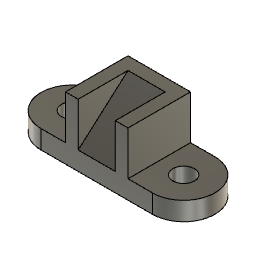
Homework - A2 (Autodesk Fusion 360 design; units mm, degrees)
Autodesk Fusion 360 part; units mm, degrees
sketch "Sketch1" plane through (0, 0, 0) normal (0, 0, 1) x (1, 0, 0)
  line L0 (-50, -30) -> (64, -30)
  line L1 (64, 34) -> (-50, 34)
  line L2 (-25, -30) -> (-25, 34)
  line L3 (39, -30) -> (39, 34)
  line L4 (-12, -30) -> (-12, 21)
  line L5 (26, -30) -> (26, 21)
  circle A0 centre (64, 2) radius 11
  circle A1 centre (-50, 2) radius 11
  line L6 (38.2512, 21) -> (39, 21) construction
  line L7 (-25, 21) -> (-24.2512, 21) construction
  line L8 (-12, 21) -> (26, 21)
  arc A2 (64, -30) -> (64, 34) centre (64, 2) ccw
  arc A3 (39, 21.975) -> (38.2512, 21) centre (64, 2) ccw
  arc A4 (-24.2512, 21) -> (-25, 21.975) centre (-50, 2) ccw
  arc A5 (-50, 34) -> (-50, -30) centre (-50, 2) ccw
  dimension "d1" = 114
  dimension "d2" = 64
  dimension "d3" = 64
  dimension "d5" = 13
  dimension "d6" = 13
  dimension "d7" = 13
  dimension "d8" = 32
  dimension "d9" = 32
  dimension "d10" = 22
  dimension "d11" = 22
  constraint horizontal L0
  constraint horizontal L1
  constraint coincident L0 L2.start
  constraint coincident L1 L2.end
  constraint perpendicular L1 L2
  constraint coincident L0 L3.start
  constraint coincident L1 L3.end
  constraint perpendicular L1 L3
  constraint coincident L0 L4.start
  constraint perpendicular L1 L4
  constraint coincident L0 L5.start
  constraint perpendicular L1 L5
  constraint coincident L2 L7.start
  constraint coincident L3 L6.end
  constraint perpendicular L3 L7
  constraint concentric A0 A2
  constraint concentric A1 A4
  constraint collinear L6 L7
  constraint collinear L7 L8
  constraint coincident L3 A3.start
  constraint concentric A2 A3
  constraint coincident L2 A4.end
  constraint concentric A4 A5
  measures "d1" distance of L0.start L0.end
  measures "d2" distance of L0.start L1.end
  measures "d3" distance of L2 L3
  measures "d5" distance of L2 L4
  measures "d6" distance of L3 L5
  measures "d7" distance of L1 L7
  measures "d8" radius of A2
  measures "d9" radius of A4
  measures "d10" diameter of A0
  measures "d11" diameter of A1
extrude "Extrude1" add sketch "Sketch1" along normal blind 64 contours L0 L1 L2 L3 L4 L5 L8
extrude "Extrude2" add sketch "Sketch1" along normal blind 19 contours L0 L1 L2 A5 | L0 L4 L5 L8 | L0 L1 L3 A2
sketch "Sketch3" plane through (-12, 0, 0) normal (1, 0, 0) x (0, 1, 0)
  line L0 (-30, 19) -> (21, 19)
  line L1 (21, 19) -> (21, 64)
  line L2 (21, 64) -> (-30, 64)
  line L3 (-30, 64) -> (-30, 19)
  line L4 (-30, 19) -> (21, 64)
  line L5 (21, 64) -> (21, 19)
  line L6 (-30, 19) -> (21, 19)
  constraint coincident L0.start L3.end
  constraint coincident L1.end L2.start
  constraint coincident L0.end L1.start
extrude "Extrude3" add sketch "Sketch3" along normal blind 38 contours L0 L1 L4 L5 L6
named bodies: "A2"
